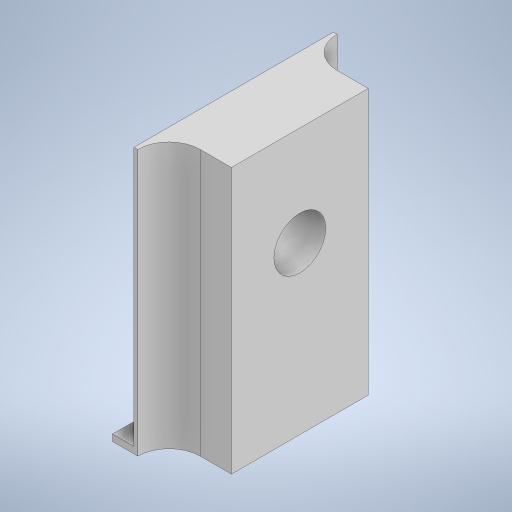
# Autodesk Inventor part: Ease of Model Bearing
Saved by Autodesk Inventor 2023 (Build 270158000, 158)
## iProperties
Created: 2023-02-26
Part Number: Ease of Model Bearing
Material: Generic
Document SubType Name: Modeling
Designer: tommy
Density: 1 g/cm^3
Appearance: Default
Author: tommy
Autodesk Inventor part; units mm, degrees
ref_plane "YZ Plane" through (0, 0, 0) normal (1, 0, 0) x (0, 1, 0)
ref_plane "XZ Plane" through (0, 0, 0) normal (0, 1, 0) x (-1, 0, 0)
ref_plane "XY Plane" through (0, 0, 0) normal (0, 0, 1) x (1, 0, 0)
sketch "Sketch1" plane through (0, 0, 0) normal (0, 1, 0) x (-1, 0, 0)
  line L0 (0, -6.4262) -> (0, -1.1938)
  arc A0 (1.1938, -1.1938) -> (2.3876, 0) centre (1.1938, 0) ccw
  arc A1 (2.3876, -7.62) -> (1.1938, -6.4262) centre (1.1938, -7.62) ccw
  line L1 (2.3876, 0) -> (2.5329, 0)
  line L2 (2.5329, 0) -> (2.5329, -7.62)
  line L3 (2.5329, -7.62) -> (2.3876, -7.62)
  line L4 (1.1938, -6.4262) -> (0, -6.4262)
  line L5 (1.1938, -1.1938) -> (0, -1.1938)
  line L6 (0, 0) -> (3.3528, 0)
  line L7 (0, -3.81) -> (2.5329, -3.81)
  line L8 (0, -7.62) -> (3.3528, -7.62)
  line L9 (3.3528, -7.62) -> (3.3528, 0)
  dimension "d2" = 2.3876
  dimension "d3" = 2.3876
  dimension "d12" = 3.3528
  constraints: 20 end point, 4 point on circle, 2 centre point, 2 horizontal, 2 midpoint, 2 symmetric about line, 2 tangent, 1 perpendicular, 1 vertical
  measures "d2" diameter of A0
  measures "d3" diameter of A1
  measures "d12" distance of L6.start L6.end
extrude "Extrusion1" add sketch "Sketch1" along normal blind 10.16 contours L0 L7 L2 L3 A1 L4 | L0 L5 A0 L1 L2 L7
sketch "Sketch2" plane through (0, 0, -1.1938) normal (1, 0, 0) x (0, 0, -1)
  circle A0 centre (2.6162, 6.35) radius 0.9922
  line L0 (0, 0) -> (5.2324, 0) projected
  point P0 (-1.1938, 0)
  dimension "d8" = 1.9844
  dimension "d9" = 6.35
  constraints: 1 centre point
  measures "d8" diameter of A0
  measures "d9" distance from line of L0 A0.centre
extrude "Extrusion3" cut sketch "Sketch2" against normal blind 127
extrude "Extrusion4" add sketch "Sketch1" along normal blind 0.254 contours L2 L6 L9 L8
body "Solid1"
